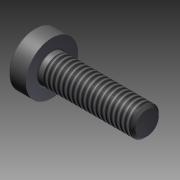
# Autodesk Inventor part: M3-10_bo
Saved by Autodesk Inventor 2011 SP1 (Build 150282100, 282)
## iProperties
Created: 2015-02-02
Part Number: M3-10_bo
Catalog Web Link: www.cadenas.de
Description: Screw_b-Couplings - Hexagon Socket Head Cap Screw
Vendor: MISUMI
Document SubType Name: Modeling
Designer: PARTuser1
Manufacturer: MISUMI
Mass: 0.108932 g
Surface Area: 1.83197 cm^2
Volume: 0.108932 cm^3
Density: 1 g/cm^3
Category: PARTsolutions
Company: MISUMI
Title: M3-10
Author: Cadenas PARTsolutions
Comments: Couplings - Hexagon Socket Head Cap Screw
PSOL_IDENT_0: {\\10.0.0.236\data_v8\23d-libs\misumi\metric\50_couplings\parts\screw_mcoc.prj},158 {VTYP=3D},{NB=M3
PSOL_IDENT_1: -10_bo},{LINA=M3-10},{NN=Screw_b},{DATE=13.11.2014 06:59:43},{GEOMDATE=04.12.2013 07:56:00},{VERSION=
PSOL_IDENT_2: },{LINEID=260},{LINESUBID=-1},{WBVAR=L}  {NB=M3-10_bo},{LINA=M3-10},{KT=DUMMY},{PN=M3-10},{M=M3},{TH
PSOL_IDENT_3: MD1=3.0000},{THMIN1=2.4590},{KK=2.00},{L=10},{LALG=10},{DK=5.5},{S=2.50},{TT=1.3},{EE=2.87},{DA=3.6}
PSOL_IDENT_4: ,{DS=3.0},{VV=0.30},{RR=0.1}
SUPPLIER: MISUMI
ARTICLENO: M3-10_bo
BOMINFO: M3-10
CREATOR: CADENAS GmbH
Autodesk Inventor part; units mm, degrees
sketch "Sketch_1" plane through (0, 0, 0) normal (0, 0, 1) x (1, 0, 0)
  line L0 (10, 0) -> (-2, 0)
  line L1 (-2, 0) -> (-2, 2.45)
  line L2 (-2, 2.45) -> (-1.7, 2.75)
  line L3 (-1.7, 2.75) -> (0, 2.75)
  line L4 (0, 2.75) -> (0, 1.6)
  arc A0 (0, 1.6) -> (0.1, 1.5) centre (0.1, 1.6) ccw
  line L5 (0.1, 1.5) -> (9.7295, 1.5)
  line L6 (9.7295, 1.5) -> (10, 1.2295)
  line L7 (10, 1.2295) -> (10, 0)
  line L8 (10, 0) -> (-2, 0)
  constraints: 18 end point, 2 point on circle, 1 centre point
revolve "Revolution1" add sketch "Sketch_1" angle 360 about axis through (10, 0, 0) along (1, 0, 0)
thread "Thread1" size "M3x0.5" class "6g" standard "ISO Metric profile" length 9.4315 offset 0.4685
sketch "Sketch_2" plane through (-2, 0, 0) normal (1, 0, 0) x (0, 0, -1)
  line L0 (-1.25, 0.7217) -> (-1.25, -0.7217)
  line L1 (-1.25, -0.7217) -> (0, -1.4434)
  line L2 (0, -1.4434) -> (1.25, -0.7217)
  line L3 (1.25, -0.7217) -> (1.25, 0.7217)
  line L4 (1.25, 0.7217) -> (0, 1.4434)
  line L5 (0, 1.4434) -> (-1.25, 0.7217)
  constraints: 12 end point
extrude "Extrusion1" cut sketch "Sketch_2" along normal blind 1.3
sketch "Sketch_5" plane through (0, 0, 0) normal (0, 0, 1) x (1, 0, 0)
  line L0 (0.0217, 0) -> (-0.7, 0)
  line L1 (-0.7, 0) -> (-0.7, 1.25)
  line L2 (-0.7, 1.25) -> (0.0217, 0)
  line L3 (0.0217, 0) -> (-0.7, 0)
  constraints: 8 end point
revolve "Revolution2" cut sketch "Sketch_5" angle 360 about axis through (0.0217, 0, 0) along (1, 0, 0)
ref_plane "SCW_XY" through (0, 0, 0) normal (1, 0, 0) x (0, 0, -1)
ref_plane "SCW_YZ" through (0, 0, 0) normal (0, 0, -1) x (0, 1, 0)
ref_plane "SCW_ZX" through (0, 0, 0) normal (0, 1, 0) x (1, 0, 0)
body "Solid1"
